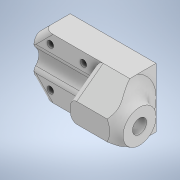
# Autodesk Inventor part: end_tip_1
Saved by Autodesk Inventor 2020 (Build 240168000, 168)
## iProperties
Created: 2019-10-27
Part Number: end_tip_1
Material: Generic
Document SubType Name: Modeling
Designer: psrob
Density: 1 g/cm^3
Appearance: Default
Author: psrob
Autodesk Inventor part; units mm, degrees
ref_plane "YZ Plane" through (0, 0, 0) normal (1, 0, 0) x (0, 1, 0)
ref_plane "XZ Plane" through (0, 0, 0) normal (0, 1, 0) x (-1, 0, 0)
ref_plane "XY Plane" through (0, 0, 0) normal (0, 0, 1) x (1, 0, 0)
sketch "Sketch1" plane through (0, 0, 0) normal (0, 0, 1) x (1, 0, 0)
  circle A0 centre (-21, -3) radius 3 projected
  line L0 (0, 0) -> (0, -6) projected
  line L1 (0, -6) -> (120, -6) projected
  line L2 (120, 0) -> (120, -6) projected
  line L3 (0, 0) -> (120, 0) projected
  line L4 (-21, -3) -> (129, -3)
  line L5 (120, -6) -> (120, -12)
  line L6 (120, -12) -> (100, -12)
  line L7 (100, -12) -> (100, 6)
  line L8 (100, 6) -> (120, 6)
  line L9 (120, 6) -> (120, -12)
  line L10 (120, -12) -> (129, -12)
  line L11 (129, -12) -> (129, 6)
  line L12 (129, 6) -> (120, 6)
  line L13 (120, 6) -> (120, -12)
  line L14 (100, -12) -> (100, -9)
  line L15 (100, -9) -> (105, -9)
  line L16 (105, -9) -> (115, -9)
  line L17 (100, 6) -> (100, 3)
  line L18 (100, 3) -> (105, 3)
  line L19 (105, 3) -> (115, 3)
  circle A1 centre (105, -9) radius 1
  circle A2 centre (115, -9) radius 1
  circle A3 centre (115, 3) radius 1
  circle A4 centre (105, 3) radius 1
  dimension "d0" = 150
  dimension "d1" = 6
  dimension "d2" = 20
  dimension "d3" = 18
  dimension "d4" = 9
  dimension "d5" = 18
  dimension "d6" = 3
  dimension "d7" = 5
  dimension "d8" = 10
  dimension "d9" = 3
  dimension "d10" = 5
  dimension "d11" = 10
  dimension "d12" = 2
  dimension "d13" = 2
  dimension "d14" = 2
  dimension "d15" = 2
  constraints: 32 end point, 4 centre point, 4 coincident, 4 parallel, 4 perpendicular, 4 point on line, 3 horizontal, 1 vertical
  measures "d0" distance of L4.start L4.end
  measures "d1" distance of L1.end L5.end
  measures "d2" distance of L7.end L8.end
  measures "d3" distance of L6.end L7.end
  measures "d4" distance of L12.end L11.end
  measures "d5" distance of L11.end L10.end
  measures "d6" distance of L6.end L14.end
  measures "d7" distance of L14.end L15.end
  measures "d8" distance of L15.end L16.end
  measures "d9" distance of L7.end L17.end
  measures "d10" distance of L17.end L18.end
  measures "d11" distance of L18.end L19.end
  measures "d12" diameter of A1
  measures "d13" diameter of A2
  measures "d14" diameter of A3
  measures "d15" diameter of A4
extrude "Extrusion1" add sketch "Sketch1" along normal blind 5 contours L7 L8 L9 L3 | L3 L2 L4 L7 | L4 L2 L1 L7 | L9 L12 L11 L4 L2 | L1 L5 L6 L7 | L4 L11 L10 L5 L2
sketch "Sketch2" plane through (0, 0, 0) normal (0, 0, -1) x (-1, 0, 0)
  line L0 (-100, -12) -> (-129, -12) projected
  line L1 (-100, 6) -> (-100, -12) projected
  line L2 (-129, 6) -> (-100, 6) projected
  line L3 (-129, -12) -> (-129, 6) projected
  circle A0 centre (-115, 3) radius 1 projected
  circle A1 centre (-105, 3) radius 1 projected
  circle A2 centre (-115, -9) radius 1 projected
  circle A3 centre (-105, -9) radius 1 projected
  line L4 (0, -6) -> (-120, -6) projected
  line L5 (0, 0) -> (-120, 0) projected
  line L6 (-120, 0) -> (-120, -6)
  point P0 (-100, 0)
  point P1 (-100, -6)
  constraints: 2 end point, 1 vertical
extrude "Extrusion2" add sketch "Sketch2" along normal blind 3 contours L0 L3 L2 L1 L5 L6 L4
sketch "Sketch3" plane through (0, 0, 5) normal (0, 0, 1) x (1, 0, 0)
  line L0 (100, -12) -> (129, -12) projected
  line L1 (129, -12) -> (129, 6) projected
  line L2 (129, 6) -> (100, 6) projected
  line L3 (100, 6) -> (100, -12) projected
  circle A0 centre (115, 3) radius 1 projected
  circle A1 centre (105, 3) radius 1 projected
  circle A2 centre (115, -9) radius 1 projected
  circle A3 centre (105, -9) radius 1 projected
  line L4 (129, -12) -> (123, -12)
  line L5 (123, -12) -> (123, 6)
  line L6 (123, 6) -> (129, 6)
  line L7 (129, 6) -> (129, -12)
  point P0 (0, 0)
  dimension "d20" = 6
  dimension "d21" = 18
  constraints: 8 end point, 2 parallel, 1 horizontal, 1 perpendicular
  measures "d20" distance of L5.end L6.end
  measures "d21" distance of L4.end L5.end
extrude "Extrusion3" add sketch "Sketch3" along normal blind 6 contours L5 L2 L1 L0
sketch "Sketch4" plane through (129, -12, -3) normal (1, 0, 0) x (0, 0, -1)
  line L0 (0, 18) -> (-14, 18) projected
  line L1 (-14, 0) -> (-14, 18) projected
  line L2 (0, 0) -> (-14, 0) projected
  line L3 (0, 18) -> (0, 0) projected
  ellipse E0 centre (-10, 203.2915) end of major axis (-13, 203.2915) minor radius 2.7456 projected
  line L4 (-10, 203.2915) -> (-10, 3.2915)
  line L5 (0, 18) -> (0, 0) projected
  line L6 (0, 9) -> (-10, 9)
  circle A0 centre (-10, 9) radius 1.5
  point P0 (-3, 12)
  dimension "d24" = 200
  dimension "d25" = 3
  constraints: 4 end point, 1 centre point, 1 coincident, 1 midpoint, 1 perpendicular, 1 point on line, 1 vertical, 1 other
  measures "d24" distance of L4.start L4.end
  measures "d25" diameter of A0
extrude "Extrusion4" cut sketch "Sketch4" against normal blind 6 contours A0 L6 L4 | L4 A0 | A0 L4 L6
thicken "Thicken1" operation add thickness 4 both sides no extend neighbours yes toward (-1, 0, 0) faces at (123, 3.4964, 7.7269)
thicken "Thicken2" operation add thickness 2 both sides no extend neighbours yes toward (0, 0, 1) faces at (122.3333, 0, 11)
sketch "Sketch5" plane through (119, -12, 5) normal (-1, 0, 0) x (0, 0, 1)
  circle A0 centre (2, 9) radius 1.5 projected
  line L0 (0, 0) -> (0, 18) projected
  line L1 (0, 0) -> (8, 0) projected
  line L2 (8, 18) -> (8, 0) projected
  line L3 (0, 18) -> (8, 18) projected
  circle A1 centre (2, 9) radius 3.5
  point P0 (-5, 12)
  dimension "d32" = 7
  constraints: 1 centre point, 1 coincident
  measures "d32" diameter of A1
extrude "Extrusion5" cut sketch "Sketch5" along normal blind 100 contours A0 | A1 L0 | L0 A1
sketch "Sketch6" plane through (119, -12, 13) normal (-1, 0, 0) x (0, 0, 1)
  circle A0 centre (-6, 9) radius 1.5 projected
  line L0 (-8, 0) -> (-8, 6.1277) projected
  line L1 (-8, 0) -> (0, 0) projected
  line L2 (0, 18) -> (0, 0) projected
  line L3 (-8, 18) -> (0, 18) projected
  line L4 (-8, 11.8723) -> (-8, 18) projected
  arc A1 (-8, 11.8723) -> (-8, 6.1277) centre (-6, 9) ccw projected
  line L5 (-8, 18) -> (0, 18) projected
  line L6 (0, 18) -> (0, 12)
  line L7 (0, 12) -> (-8, 18)
  line L8 (0, 18) -> (0, 0) projected
  line L9 (0, 0) -> (0, 6)
  line L10 (0, 6) -> (-8, 0)
  point P0 (-13, 12)
  dimension "d35" = 6
  dimension "d36" = 6
  constraints: 8 end point, 2 point on line
  measures "d35" distance of L2.start L6.end
  measures "d36" distance of L1.end L9.end
extrude "Extrusion6" cut sketch "Sketch6" against normal blind 100 contours L10 L2 L1 | L7 L3 L2
sketch "Sketch7" plane through (129, -12, -3) normal (1, 0, 0) x (0, 0, -1)
  circle A0 centre (-10, 9) radius 1.5 projected
  line L0 (-16, 6) -> (-8, 0) projected
  line L1 (0, 0) -> (-8, 0) projected
  line L2 (0, 18) -> (0, 0) projected
  line L3 (0, 18) -> (-8, 18) projected
  line L4 (-8, 18) -> (-16, 12) projected
  line L5 (-16, 6) -> (-16, 12) projected
  circle A1 centre (-10, 9) radius 2.15
  circle A2 centre (-10, 9) radius 5
  point P0 (-3, 12)
  dimension "d39" = 4.3
  dimension "d40" = 10
  constraints: 2 centre point, 2 coincident
  measures "d39" diameter of A1
  measures "d40" diameter of A2
extrude "Extrusion7" add sketch "Sketch7" along normal blind 5 contours A2
fillet "Fillet1" radius 5 1 edges at (129, -3, 12)
fillet "Fillet2" radius 2 2 edges at (119, 3, 9) (119, -9, 9)
fillet "Fillet3" radius 2 2 edges at (109.5, -0.1277, 5) (109.5, -5.8723, 5)
chamfer "Chamfer1" distance 3 angle 45 2 edges at (100, 6, 1) (100, -12, 1)
fillet "Fillet4" radius 2 2 edges at (101.5, 4.5, 5) (101.5, -10.5, 5)
body "Solid1"
